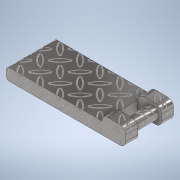
# Autodesk Inventor part: Pedals
Saved by Autodesk Inventor 2022 (Build 260153000, 153)
## iProperties
Created: 2021-12-07
Part Number: Pedals
Material: Generic
Document SubType Name: Modeling
Designer: Vedic
Density: 1 g/cm^3
Appearance: Default
Author: Vedic
Autodesk Inventor part; units mm, degrees
ref_plane "YZ Plane" through (0, 0, 0) normal (1, 0, 0) x (0, 1, 0)
ref_plane "XZ Plane" through (0, 0, 0) normal (0, 1, 0) x (-1, 0, 0)
ref_plane "XY Plane" through (0, 0, 0) normal (0, 0, 1) x (1, 0, 0)
sketch "Sketch1" plane through (0, 0, 0) normal (0, 1, 0) x (-1, 0, 0)
  line L0 (35.2615, 31.9433) -> (-167.9385, 31.9433)
  line L1 (-167.9385, 31.9433) -> (-167.9385, -69.6567)
  line L2 (-167.9385, -69.6567) -> (35.2615, -69.6567)
  line L3 (35.2615, -69.6567) -> (35.2615, 31.9433)
  line L4 (-167.9385, 31.9433) -> (-218.7385, 31.9433)
  line L5 (-218.7385, 31.9433) -> (-218.7385, 6.5433)
  line L6 (-218.7385, 6.5433) -> (-167.9385, 6.5433)
  line L7 (-167.9385, 6.5433) -> (-167.9385, 31.9433)
  line L8 (-167.9385, -69.6567) -> (-218.7385, -69.6567)
  line L9 (-218.7385, -69.6567) -> (-218.7385, -44.2567)
  line L10 (-218.7385, -44.2567) -> (-167.9385, -44.2567)
  line L11 (-167.9385, -44.2567) -> (-167.9385, -69.6567)
  point P0 (0, 0)
  point P1 (-167.9385, 6.5433)
  dimension "d0" = 101.6
  dimension "d1" = 203.2
  dimension "d2" = 50.8
  dimension "d3" = 50.8
  constraints: 24 end point, 6 parallel, 3 horizontal, 3 perpendicular, 1 collinear, 1 point on line
  measures "d0" distance of L2.end L0.start
  measures "d1" distance of L0.start L0.end
  measures "d2" distance between parallel lines of L1 L5
  measures "d3" distance between parallel lines of L10 L6
extrude "Extrusion1" add sketch "Sketch1" along normal blind 38.1 contours L1 L6 L5 L4 | L8 L9 L10 L1
extrude "Extrusion2" add sketch "Sketch1" along normal blind 25.4 contours L3 L2 L1 L0
sketch "Sketch2" plane through (167.9385, 38.1, 31.9433) normal (0, 0, 1) x (1, 0, 0)
  line L0 (50.8, -38.1) -> (50.8, 0) construction
  line L1 (0, 0) -> (50.8, 0) construction
  line L2 (50.8, -19.05) -> (31.75, -19.05) construction
  line L3 (31.75, -19.05) -> (31.75, 0) construction
  line L4 (31.75, 0) -> (50.8, 0) construction
  line L5 (50.8, 0) -> (50.8, -19.05) construction
  circle A0 centre (31.75, -19.05) radius 12.7
  point P0 (-167.9385, -38.1)
  dimension "d8" = 25.4
  constraints: 8 end point, 2 parallel, 2 perpendicular, 1 centre point, 1 coincident, 1 horizontal, 1 midpoint, 1 point on line
  measures "d8" diameter of A0
extrude "Extrusion3" add sketch "Sketch2" against normal through all
fillet "Fillet1" radius 12.7 6 edges at (167.9385, 38.1, 19.2433) (167.9385, 38.1, -56.9567) (218.7385, 38.1, 19.2433) (218.7385, 38.1, -56.9567) (218.7385, 0, 19.2433) (218.7385, 0, -56.9567)
fillet "Fillet2" radius 6.35 2 edges at (-35.2615, 25.4, -18.8567) (-35.2615, 0, -18.8567)
body "Solid1"
